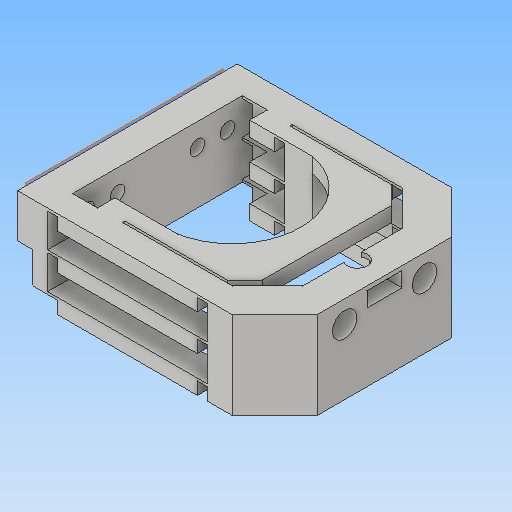
# Autodesk Inventor part: cellSTORM_v5_focussingunit_1
Saved by Autodesk Inventor 2019.4 (Build 234330000, 330)
## iProperties
Created: 2020-04-26
Part Number: cellSTORM_v5_focussingunit_1
Material: Generic
Document SubType Name: Modeling
Designer: diederichbenedict
Density: 1 g/cm^3
Appearance: Default
Mass: 20.2121 g
Surface Area: 144.301 cm^2
Volume: 20.2121 cm^3
Author: diederichbenedict
Autodesk Inventor part; units mm, degrees
ref_plane "YZ Plane" through (0, 0, 0) normal (1, 0, 0) x (0, 1, 0)
ref_plane "XZ Plane" through (0, 0, 0) normal (0, 1, 0) x (-1, 0, 0)
ref_plane "XY Plane" through (0, 0, 0) normal (0, 0, 1) x (1, 0, 0)
ref_plane "Work Plane1" through (-20.9765, 40.8646, -17.35) normal (-1, 0, 0) x (0, 1, 0)
sketch "Sketch1" plane through (-20.9765, 32.0794, -17.35) normal (1, 0, 0) x (0, -1, 0)
  line L0 (2.0794, -30.35) -> (-37.9206, -30.35)
  line L1 (2.0794, -30.35) -> (-37.9206, -30.35) construction
  line L2 (2.0794, -4.35) -> (-37.9206, -4.35) construction
  line L3 (-55.6353, -17.35) -> (78.0542, -17.35) construction
  circle A0 centre (-4.5, -4.35) radius 3.25 construction
  circle A1 centre (-4.5, -30.35) radius 3.25 construction
  line L4 (0, -36) -> (-9, -36) construction
  line L5 (0, 0) -> (0, -36) construction
  line L6 (-9, 0) -> (0, 0) construction
  line L7 (-9, 0) -> (-9, -36) construction
  line L8 (-0.15, -17.35) -> (-8.85, -17.35)
  line L9 (-8.85, -17.35) -> (-8.85, 4.65)
  line L10 (-8.85, 4.65) -> (-0.15, 4.65)
  line L11 (-0.15, 4.65) -> (-0.15, -17.35)
  point P0 (32.0794, -17.35)
  dimension "d0" = 22
  dimension "d1" = 0.15
  dimension "d2" = 0.15
  constraints: 16 end point, 5 horizontal, 2 parallel, 1 perpendicular, 1 point on line, 6 other
  measures "d0" distance of L8.end L9.end
  measures "d1" distance between parallel lines of L5 L11
  measures "d2" distance between parallel lines of L9 L7
extrude "Extrusion1" add sketch "Sketch1" along normal blind 4
sketch "Sketch2" plane through (-16.9765, 32.0794, -17.35) normal (1, 0, 0) x (0, 0, -1)
  line L0 (-17.35, 8.85) -> (-17.35, 0.15) projected
  line L1 (-17.35, 0.15) -> (4.65, 0.15) projected
  line L2 (4.65, 0.15) -> (4.65, 8.85) projected
  line L3 (4.65, 8.85) -> (-17.35, 8.85) projected
  line L4 (4.65, 0.15) -> (4.65, 8.85) projected
  line L5 (4.65, 8.85) -> (-17.35, 8.85)
  line L6 (-17.35, 8.85) -> (-17.35, -13.8794)
  line L7 (-17.35, -13.8794) -> (4.65, -13.8794)
  line L8 (4.65, -13.8794) -> (4.65, 8.85)
  line L9 (-32, -17.0794) -> (0, -17.0794) projected
  line L10 (-32, -14.0794) -> (0, -14.0794) projected
  point P0 (-17.35, -32.0794)
  dimension "d47" = 0.2
  constraints: 8 end point, 2 parallel, 1 horizontal, 1 perpendicular
  measures "d47" distance between parallel lines of L10 L7
extrude "Extrusion2" add sketch "Sketch2" along normal blind 2 and the other way blind 1
sketch "Sketch3" plane through (-20.9765, 32.2294, -22) normal (0, 0, -1) x (-1, 0, 0)
  line L0 (0, 8.7) -> (0, 0) projected
  line L1 (0, 8.7) -> (-6, 8.7) projected
  line L2 (-6, -14.0294) -> (-6, 8.7) projected
  line L3 (-3, -14.0294) -> (-6, -14.0294) projected
  line L4 (-3, 0) -> (-3, -14.0294) projected
  line L5 (0, 0) -> (-3, 0) projected
  line L6 (-6, 8.7) -> (-8, 8.7)
  line L7 (-8, 8.7) -> (-8, 8.2)
  line L8 (-8, 8.2) -> (-6, 8.2)
  line L9 (-6, 8.2) -> (-6, 8.7)
  line L10 (-6, 1.45) -> (-8, 1.45)
  line L11 (-8, 1.45) -> (-8, 0.95)
  line L12 (-8, 0.95) -> (-6, 0.95)
  line L13 (-6, 0.95) -> (-6, 1.45)
  line L14 (-8, -6.3) -> (-8, -5.8)
  line L15 (-6, -13.5294) -> (-6, -14.0294)
  line L16 (-8, 8.7) -> (-36, 8.7)
  line L17 (-36, 8.7) -> (-36, 5.7)
  line L18 (-36, 5.7) -> (-8, 5.7)
  line L19 (-8, 5.7) -> (-8, 8.7)
  line L20 (-8, 1.45) -> (-36, 1.45)
  line L21 (-36, 1.45) -> (-36, -1.55)
  line L22 (-36, -1.55) -> (-8, -1.55)
  line L23 (-8, -1.55) -> (-8, 1.45)
  line L24 (-8, -5.8) -> (-36, -5.8)
  line L25 (-36, -5.8) -> (-36, -8.8)
  line L26 (-36, -8.8) -> (-8, -8.8)
  line L27 (-8, -8.8) -> (-8, -5.8)
  line L28 (-36, -5.8) -> (-38, -5.8)
  line L29 (-38, -5.8) -> (-38, -6.3)
  line L30 (-38, -6.3) -> (-36, -6.3)
  line L31 (-36, -6.3) -> (-36, -5.8)
  line L32 (-36, 1.45) -> (-38, 1.45)
  line L33 (-38, 1.45) -> (-38, 0.95)
  line L34 (-38, 0.95) -> (-36, 0.95)
  line L35 (-36, 0.95) -> (-36, 1.45)
  line L36 (-36, 8.7) -> (-38, 8.7)
  line L37 (-38, 8.7) -> (-38, 8.2)
  line L38 (-38, 8.2) -> (-36, 8.2)
  line L39 (-36, 8.2) -> (-36, 8.7)
  line L40 (-38, 8.7) -> (-43, 8.7)
  line L41 (-43, 8.7) -> (-43, -8.8)
  line L42 (-43, -8.8) -> (-38, -8.8)
  line L43 (-38, -8.8) -> (-38, 8.7)
  line L44 (-8, -5.8) -> (-6, -5.8)
  line L45 (-6, -5.8) -> (-6, -6.3)
  line L46 (-6, -6.3) -> (-8, -6.3)
  line L47 (-8, -6.3) -> (-8, -5.8)
  point P0 (-20.9765, -32.2294)
  dimension "d8" = 2
  dimension "d9" = 0.5
  dimension "d10" = 2
  dimension "d11" = 0.5
  dimension "d12" = 0.5
  dimension "d13" = 7.25
  dimension "d14" = 28
  dimension "d15" = 3
  dimension "d16" = 28
  dimension "d17" = 3
  dimension "d18" = 28
  dimension "d19" = 3
  dimension "d20" = 2
  dimension "d21" = 0.5
  dimension "d22" = 2
  dimension "d23" = 0.5
  dimension "d24" = 0.5
  dimension "d25" = 5
  dimension "d48" = 14.5
  constraints: 84 end point, 21 parallel, 10 horizontal, 10 perpendicular, 5 point on line
  measures "d8" distance of L8.end L7.end
  measures "d9" distance of L7.end L6.end
  measures "d10" distance of L12.end L11.end
  measures "d11" distance of L11.end L10.end
  measures "d12" distance of L14.start L14.end
  measures "d13" distance between parallel lines of L10 L1
  measures "d14" distance of L18.end L17.end
  measures "d15" distance of L17.end L16.end
  measures "d16" distance of L22.end L21.end
  measures "d17" distance of L21.end L20.end
  measures "d18" distance of L26.end L25.end
  measures "d19" distance of L25.end L24.end
  measures "d20" distance of L30.end L29.end
  measures "d21" distance of L29.end L28.end
  measures "d22" distance of L34.end L33.end
  measures "d23" distance of L33.end L32.end
  measures "d24" distance of L37.end L36.end
  measures "d25" distance of L42.end L41.end
  measures "d48" distance between parallel lines of L24 L1
extrude "Extrusion3" add sketch "Sketch3" against normal blind 5 contours L2 L8 L7 L6 | L7 L19 L18 L17 L16 | L2 L12 L11 L10 | L17 L38 L37 L36 | L11 L23 L22 L21 L20 | L37 L43 L33 L29 L42 L41 L40 | L2 L46 L14 L44 | L21 L34 L33 L32 | L14 L27 L26 L25 L24 | L25 L30 L29 L28
sketch "Sketch4" plane through (-20.9765, 32.2294, -17) normal (0, 0, 1) x (1, 0, 0)
  line L0 (23.4765, -14.7269) -> (23.4765, -52.3718) construction
  line L1 (18.4765, -14.7269) -> (18.4765, -47.4664) construction
  line L2 (20.9765, -32.2294) -> (20.9765, -11.9231) construction
  line L3 (6, -6.3) -> (6, -5.8) construction
  line L4 (8, -6.3) -> (8, -8.8) construction
  line L5 (8, -8.8) -> (36, -8.8) construction
  line L6 (36, -8.8) -> (36, -6.3) construction
  line L7 (36, -6.3) -> (38, -6.3) construction
  line L8 (38, -6.3) -> (38, -8.8) construction
  line L9 (38, -8.8) -> (43, -8.8) construction
  line L10 (43, -8.8) -> (43, 8.7) construction
  line L11 (43, 8.7) -> (6, 8.7) construction
  line L12 (6, 8.2) -> (6, 8.7) construction
  line L13 (6, 8.2) -> (8, 8.2) construction
  line L14 (8, 8.2) -> (8, 5.7) construction
  line L15 (8, 5.7) -> (36, 5.7) construction
  line L16 (36, 5.7) -> (36, 8.2) construction
  line L17 (36, 8.2) -> (38, 8.2) construction
  line L18 (38, 8.2) -> (38, 1.45) construction
  line L19 (38, 1.45) -> (6, 1.45) construction
  line L20 (6, 0.95) -> (6, 1.45) construction
  line L21 (6, 0.95) -> (8, 0.95) construction
  line L22 (8, 0.95) -> (8, -1.55) construction
  line L23 (8, -1.55) -> (36, -1.55) construction
  line L24 (36, -1.55) -> (36, 0.95) construction
  line L25 (36, 0.95) -> (38, 0.95) construction
  line L26 (38, 0.95) -> (38, -5.8) construction
  line L27 (36, -8.8) -> (8, -8.8) construction
  line L28 (10.9765, -8.8) -> (15.9765, -8.8) construction
  line L29 (15.9765, -8.8) -> (15.9765, -5.8) construction
  line L30 (15.9765, -5.8) -> (10.9765, -5.8) construction
  line L31 (10.9765, -5.8) -> (10.9765, -8.8) construction
  line L32 (10.9765, -8.8) -> (15.9765, -8.8)
  line L33 (15.9765, -8.8) -> (15.9765, -5.8)
  line L34 (15.9765, -5.8) -> (10.9765, -5.8)
  line L35 (10.9765, -5.8) -> (10.9765, -8.8)
  line L36 (36, -1.55) -> (8, -1.55) projected
  line L37 (38, 1.45) -> (6, 1.45) projected
  line L38 (10.9765, -1.55) -> (15.9765, -1.55)
  line L39 (15.9765, -1.55) -> (15.9765, 1.45)
  line L40 (15.9765, 1.45) -> (10.9765, 1.45)
  line L41 (10.9765, 1.45) -> (10.9765, -1.55)
  line L42 (36, 5.7) -> (8, 5.7) projected
  line L43 (43, 8.7) -> (6, 8.7) projected
  line L44 (10.9765, 5.7) -> (15.9765, 5.7)
  line L45 (15.9765, 5.7) -> (15.9765, 8.7)
  line L46 (15.9765, 8.7) -> (10.9765, 8.7)
  line L47 (10.9765, 8.7) -> (10.9765, 5.7)
  line L48 (38, -5.8) -> (6, -5.8) projected
  line L49 (6, -6.3) -> (8, -6.3) projected
  line L50 (38, -5.8) -> (6, -5.8) projected
  dimension "d28" = 5
  dimension "d29" = 5
  constraints: 38 end point, 8 parallel, 8 point on line, 4 horizontal, 4 perpendicular, 3 vertical, 4 other
  measures "d28" distance of L30.end L29.end
  measures "d29" distance between parallel lines of L29 L2
extrude "Extrusion4" add sketch "Sketch4" along normal blind 0.5
sketch "Sketch5" plane through (-20.9765, 32.2294, -16.5) normal (0, 0, 1) x (1, 0, 0)
  line L0 (10.9765, -8.8) -> (15.9765, -8.8) projected
  line L1 (15.9765, -8.8) -> (15.9765, -5.8) projected
  line L2 (15.9765, -5.8) -> (10.9765, -5.8) projected
  line L3 (10.9765, -5.8) -> (10.9765, -8.8) projected
  line L4 (10.9765, -1.55) -> (15.9765, -1.55) projected
  line L5 (15.9765, -1.55) -> (15.9765, 1.45) projected
  line L6 (15.9765, 1.45) -> (10.9765, 1.45) projected
  line L7 (10.9765, 1.45) -> (10.9765, -1.55) projected
  line L8 (10.9765, 5.7) -> (15.9765, 5.7) projected
  line L9 (15.9765, 5.7) -> (15.9765, 8.7) projected
  line L10 (15.9765, 8.7) -> (10.9765, 8.7) projected
  line L11 (10.9765, 8.7) -> (10.9765, 5.7) projected
  line L12 (15.9765, -5.8) -> (17.9765, -5.8)
  line L13 (17.9765, -5.8) -> (17.9765, -6.3)
  line L14 (17.9765, -6.3) -> (15.9765, -6.3)
  line L15 (15.9765, -6.3) -> (15.9765, -5.8)
  line L16 (15.9765, 1.45) -> (17.9765, 1.45)
  line L17 (17.9765, 1.45) -> (17.9765, 0.95)
  line L18 (17.9765, 0.95) -> (15.9765, 0.95)
  line L19 (15.9765, 0.95) -> (15.9765, 1.45)
  line L20 (15.9765, 8.7) -> (17.9765, 8.7)
  line L21 (17.9765, 8.7) -> (17.9765, 8.2)
  line L22 (17.9765, 8.2) -> (15.9765, 8.2)
  line L23 (15.9765, 8.2) -> (15.9765, 8.7)
  line L24 (23.4765, -14.7269) -> (23.4765, -52.3718)
  line L25 (18.4765, -14.7269) -> (18.4765, -47.4664)
  line L26 (36, -8.8) -> (8, -8.8) projected
  line L27 (23.4765, -8.8) -> (17.9765, -8.8)
  line L28 (17.9765, -8.8) -> (17.9765, 8.7)
  line L29 (17.9765, 8.7) -> (23.4765, 8.7)
  line L30 (23.4765, 8.7) -> (23.4765, -8.8)
  line L31 (23.4765, -8.8) -> (17.9765, -8.8)
  line L32 (17.9765, -8.8) -> (17.9765, -10.8)
  line L33 (17.9765, -10.8) -> (23.4765, -10.8)
  line L34 (23.4765, -10.8) -> (23.4765, -8.8)
  point P0 (20.9765, -32.2294)
  dimension "d32" = 2
  dimension "d33" = 0.5
  dimension "d34" = 0.5
  dimension "d35" = 0.5
  dimension "d38" = 2
  constraints: 44 end point, 10 parallel, 5 horizontal, 5 perpendicular, 2 point on line, 2 vertical, 4 other
  measures "d32" distance of L13.end L14.end
  measures "d33" distance of L12.end L13.end
  measures "d34" distance of L16.end L17.end
  measures "d35" distance of L20.end L21.end
  measures "d38" distance of L32.end L31.end
extrude "Extrusion5" add sketch "Sketch5" along normal blind 3 contours L3 L2 L1 L0 | L1 L12 L13 L14 | L28 L13 L17 L21 L29 L30 L26 | L26 L34 L33 L32 | L18 L5 L16 L17 | L21 L22 L9 L20 | L5 L4 L7 L6 | L9 L8 L11 L10
sketch "Sketch6" plane through (-3, 40.9294, -17.5) normal (0, -1, 0) x (1, 0, 0)
  circle A0 centre (3, 17.5) radius 10 construction
  circle A1 centre (3, 17.5) radius 13 construction
  line L0 (-2, 1) -> (-2, 4) projected
  line L1 (0, 1) -> (0, 4) projected
  line L2 (0, 1) -> (5.5, 1) projected
  line L3 (0, 4) -> (5.5, 4) projected
  line L4 (5.5, 1) -> (5.5, 4) projected
  line L5 (5.5, 1) -> (18.5, 1)
  line L6 (-9.9765, 0.5) -> (18.0235, 0.5) projected
  line L7 (5.5, 1) -> (18.5, 1) construction
  line L8 (0, 1) -> (0, 4) projected
  line L9 (0, 4) -> (-0.165, 4.165)
  line L10 (0, 4) -> (1, 4) construction
  line L11 (0, 4) -> (-7, 4) construction
  line L12 (0, 4.8509) -> (0, 1) construction
  line L13 (-2, 1) -> (0, 1) construction
  line L14 (0, 1) -> (5.5, 1) construction
  line L15 (5.5, 1) -> (18.5, 1)
  line L16 (18.5017, 17.5) -> (16.7295, 17.5)
  line L17 (18.5017, 17.5) -> (16.7295, 17.5)
  line L18 (18.5, 1) -> (22.0235, 4.5235)
  line L19 (18.5, 1) -> (23.483, 1) construction
  line L20 (25.0235, -4.5) -> (25.0235, 0.5) projected
  line L21 (22.0235, 4.5235) -> (22.0235, 17.5)
  line L22 (22.0235, 17.5) -> (18.5017, 17.5)
  line L23 (-8.7686, 17.5) -> (-8.4695, 17.5)
  line L24 (-8.4695, 17.5) -> (-8.4695, 6.7071)
  arc A2 (-8.7686, 17.5) -> (-8.4695, 14.8636) centre (3, 17.5) ccw
  arc A3 (-0.165, 4.165) -> (0, 4.1269) centre (3, 17.5) ccw
  arc A4 (5.5, 4) -> (16.7295, 17.5) centre (3, 17.5) ccw
  point P0 (-2, 0.5)
  point P1 (13, 17.5)
  point P2 (-10, 17.5)
  point P3 (-7, 17.5)
  dimension "d39" = 13
  dimension "d40" = 0
  dimension "d42" = 135
  dimension "d109" = 0
  dimension "d110" = 45
  dimension "d133" = 3
  constraints: 31 end point, 10 point on circle, 4 collinear, 4 horizontal, 3 centre point, 2 equal length, 2 parallel, 2 perpendicular, 2 point on line, 1 coincident, 1 vertical
  measures "d39" distance of L2.end L5.end
  measures "d40" distance between parallel lines of L7 L5
  measures "d42" angle of L10 L9
  measures "d109" distance from line of A2.centre L16
  measures "d110" angle of L19 L18
  measures "d133" distance between parallel lines of L21 L20
extrude "Extrusion6" add sketch "Sketch6" along normal up to surface (3 mm away) contours L1 L3 L4 L2 | L4 A4 L16 L22 L21 L18 L5
sketch "Sketch8" plane through (17.0235, 23.4294, -22) normal (0, -1, 0) x (1, 0, 0)
  line L0 (5, 0) -> (0, 0) projected
  line L1 (5, 0) -> (5, 5) projected
  line L2 (0, 5) -> (5, 5) projected
  line L3 (0, 0) -> (0, 5) projected
  line L4 (0, 5) -> (7.0711, 12.0711)
  line L5 (0, 5) -> (10, 5) construction
  line L6 (5, 0) -> (13.4853, 8.4853)
  line L7 (5, 0) -> (17, 0) construction
  line L8 (13.4853, 8.4853) -> (13.4853, 25)
  line L9 (13.4853, 25) -> (7.0711, 25)
  line L10 (7.0711, 25) -> (7.0711, 12.0711)
  point P0 (-17.0235, 22)
  point P1 (-1.5235, 25)
  dimension "d_1" = 10
  dimension "d55" = 45
  dimension "d56" = 12
  constraints: 14 end point, 2 equal length, 2 horizontal, 2 perpendicular, 1 parallel, 1 point on line, 1 vertical
  measures "d_1" distance of L2.start L4.end
  measures "d55" angle of L5 L4
  measures "d56" distance of L0.start L6.end
extrude "Extrusion8" add sketch "Sketch8" against normal up to surface (17.5 mm away)
sketch "Sketch21" plane through (-14.9765, 37.9294, 0) normal (1, 0, 0) x (0, 1, 0)
  line L0 (-5.7, -22) -> (-5.7, 0) projected
  line L1 (3, 0) -> (3, -22) projected
  circle A0 centre (-1.4574, -8) radius 1.45
  circle A1 centre (-1.4574, -14) radius 1.45
  line L2 (-5.7, 0) -> (3, 0) projected
  line L3 (3, -22) -> (-5.7, -22) projected
  point P0 (-37.9294, 0)
  dimension "d112" = 2.9
  dimension "d113" = 2.9
  dimension "d114" = 8
  dimension "d115" = 8
  constraints: 2 centre point
  measures "d112" diameter of A0
  measures "d113" diameter of A1
  measures "d114" distance from line of A0.centre L2
  measures "d115" distance from line of A1.centre L3
extrude "Extrusion20" cut sketch "Sketch21" against normal through all contours A0 | A1
mirror "Mirror3" about plane through (-20.9765, 40.9294, 0) normal (0, 0, 1) of "Extrusion1", "Extrusion2", "Extrusion3", "Extrusion4", "Extrusion5", "Extrusion6", "Extrusion8", "Extrusion20"
sketch "Sketch22" plane through (30.5088, 23.4294, -13.5147) normal (1, 0, 0) x (0, 0, -1)
  circle A0 centre (-5.5147, 13.0426) radius 1.45 projected
  circle A1 centre (-21.5147, 13.0426) radius 1.45 projected
  circle A2 centre (-5.5147, 13.0426) radius 2.45
  circle A3 centre (-21.5147, 13.0426) radius 2.45
  point P0 (-13.5147, -23.4294)
  dimension "d118" = 1
  dimension "d119" = 1
  constraints: 2 centre point
  measures "d118" radial gap between concentric circles of A0 A2
  measures "d119" radial gap between concentric circles of A1 A3
extrude "Extrusion21" cut sketch "Sketch22" against normal blind 10 contours A0 | A1 | A2 | A3
sketch "Sketch23" plane through (-20.9765, 40.9294, -22) normal (0, 1, 0) x (1, 0, 0)
  line L0 (51.4853, -8.4853) -> (51.4853, -35.5147) projected
  line L1 (43, 0) -> (51.4853, -8.4853) projected
  line L2 (0, 0) -> (43, 0) projected
  line L3 (0, -44) -> (0, 0) projected
  line L4 (0, -44) -> (43, -44) projected
  line L5 (43, -44) -> (51.4853, -35.5147) projected
  line L6 (6, -5) -> (6, -39) projected
  line L7 (10.9765, -5) -> (6, -5) projected
  line L8 (10.9765, -5) -> (10.9765, -8.5) projected
  line L9 (10.9765, -39) -> (10.9765, -35.5) projected
  line L10 (10.9765, -39) -> (6, -39) projected
  line L11 (45.0711, -12.0711) -> (45.0711, -31.9289) projected
  line L12 (45.0711, -31.9289) -> (38, -39) projected
  line L13 (38, -39) -> (15.9765, -39) projected
  line L14 (15.9765, -39) -> (15.9765, -38.5) projected
  line L15 (36.4765, -38.5) -> (15.9765, -38.5) projected
  line L16 (36.4765, -5.5) -> (15.9765, -5.5) projected
  line L17 (15.9765, -5) -> (15.9765, -5.5) projected
  line L18 (38, -5) -> (15.9765, -5) projected
  line L19 (45.0711, -12.0711) -> (38, -5) projected
  circle A0 centre (46.0711, -22) radius 2
  line L20 (45.0711, -12.0711) -> (45.0711, -31.9289) projected
  line L21 (40, -34.9765) -> (36.4765, -38.5) projected
  line L22 (40, -34.9765) -> (40, -9.0235) projected
  line L23 (40, -9.0235) -> (36.4765, -5.5) projected
  line L24 (23.4765, -8.5) -> (10.9765, -8.5) projected
  arc A1 (23.4765, -35.5) -> (23.4765, -8.5) centre (20.9765, -22) ccw projected
  line L25 (23.4765, -35.5) -> (10.9765, -35.5) projected
  point P0 (20.9765, -22)
  dimension "d122" = 4
  dimension "d123" = 1
  dimension "d124" = 0
  constraints: 1 centre point
  measures "d122" diameter of A0
  measures "d123" distance from line of A0.centre L20
  measures "d124" vertical distance of A0.centre point (20.976, -22)
extrude "Extrusion22" cut sketch "Sketch23" against normal through all contours A0 L11 | L11 A0
sketch "Sketch24" plane through (-12.9765, 23.4294, 22) normal (0, 0, 1) x (1, 0, 0)
  line L0 (-8, 17.5) -> (35, 17.5) projected
  line L1 (-8, 17.5) -> (-8, 8.8) projected
  line L2 (-8, 8.8) -> (-5, 8.8) projected
  line L3 (-5, 8.8) -> (-5, -5.2294) projected
  line L4 (-5, -5.2294) -> (-2, -5.2294) projected
  line L5 (-2, -5.2294) -> (-2, 2.5) projected
  line L6 (0, 2.5) -> (-2, 2.5) projected
  line L7 (0, 0) -> (0, 2.5) projected
  line L8 (28, 0) -> (0, 0) projected
  line L9 (28, 2.5) -> (28, 0) projected
  line L10 (30, 2.5) -> (28, 2.5) projected
  line L11 (30, 0) -> (30, 2.5) projected
  line L12 (35, 0) -> (30, 0) projected
  line L13 (35, 17.5) -> (35, 0) projected
  line L14 (-2, 3) -> (-2, 9.75) projected
  line L15 (0, 9.75) -> (-2, 9.75) projected
  line L16 (0, 7.25) -> (0, 9.75) projected
  line L17 (28, 7.25) -> (0, 7.25) projected
  line L18 (28, 9.75) -> (28, 7.25) projected
  line L19 (30, 9.75) -> (28, 9.75) projected
  line L20 (30, 3) -> (30, 9.75) projected
  line L21 (-2, 3) -> (30, 3) projected
  line L22 (0, 17) -> (-2, 17) projected
  line L23 (0, 14.5) -> (0, 17) projected
  line L24 (28, 14.5) -> (0, 14.5) projected
  line L25 (28, 17) -> (28, 14.5) projected
  line L26 (30, 17) -> (28, 17) projected
  line L27 (30, 10.25) -> (30, 17) projected
  line L28 (-2, 10.25) -> (30, 10.25) projected
  line L29 (-2, 10.25) -> (-2, 17) projected
  line L30 (-5, -5.2294) -> (-2, -5.2294) projected
  line L31 (-5, 8.8) -> (-5, -5.2294) projected
  line L32 (-2, -5.2294) -> (-5, -5.2294)
  line L33 (-5, -5.2294) -> (-5, 2.5)
  line L34 (-5, 2.5) -> (-2, 2.5)
  line L35 (-2, 2.5) -> (-2, -5.2294)
  point P0 (12.9765, -23.4294)
  constraints: 8 end point, 2 parallel, 1 horizontal, 1 perpendicular, 1 point on line
extrude "Extrusion23" cut sketch "Sketch24" against normal through all contours L34 L5 L4 L3
sketch "Sketch25" plane through (24.0946, 23.4294, 9.9289) normal (-1, 0, 0) x (0, 0, 1)
  line L0 (-8.1969, 17.5) -> (-8.1969, 0) projected
  line L1 (-11.661, 0) -> (-11.661, 17.5) projected
  line L2 (-6.4289, 16.6633) -> (-13.4289, 16.6633)
  line L3 (-13.4289, 16.6633) -> (-13.4289, 13.6633)
  line L4 (-13.4289, 13.6633) -> (-6.4289, 13.6633)
  line L5 (-6.4289, 13.6633) -> (-6.4289, 16.6633)
  line L6 (-6.4289, 16.6633) -> (-13.4289, 13.6633) construction
  line L7 (-13.4289, 16.6633) -> (-6.4289, 13.6633) construction
  point P0 (-9.9289, -23.4294)
  point P1 (-9.9289, 15.1633)
  dimension "d129" = 7
  dimension "d130" = 3
  constraints: 12 end point, 2 midpoint, 2 parallel, 1 horizontal, 1 perpendicular
  measures "d129" distance of L4.end L3.end
  measures "d130" distance of L3.end L2.end
extrude "Extrusion24" cut sketch "Sketch25" against normal through all
body "Solid1"
